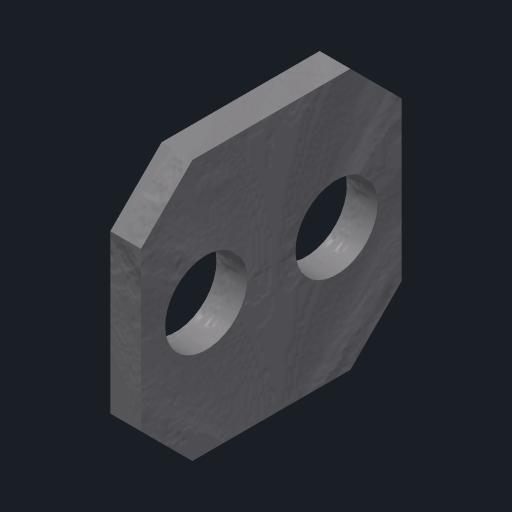
# Autodesk Inventor part: ACOPLE_TORNILLO_DOBLE
Saved by Autodesk Inventor 2024.3 (Build 283343000, 343)
## iProperties
Created: 2024-06-02
Part Number: ACOPLE_TORNILLO_DOBLE
Material: Steel, Mild, Welded
Document SubType Name: Modeling
Designer: Niler
Density: 7.85 g/cm^3
Appearance: Weld - Steel Mild
Author: Niler
Autodesk Inventor part; units mm, degrees
ref_plane "YZ Plane" through (0, 0, 0) normal (1, 0, 0) x (0, 1, 0)
ref_plane "XZ Plane" through (0, 0, 0) normal (0, 1, 0) x (-1, 0, 0)
ref_plane "XY Plane" through (0, 0, 0) normal (0, 0, 1) x (1, 0, 0)
sketch "Sketch1" plane through (0, 0, 0) normal (1, 0, 0) x (0, 1, 0)
  line L0 (-12.7, 12.7) -> (12.7, 12.7)
  line L1 (12.7, 12.7) -> (12.7, -12.7)
  line L2 (12.7, -12.7) -> (-12.7, -12.7)
  line L3 (-12.7, -12.7) -> (-12.7, 12.7)
  line L4 (-12.7, 12.7) -> (12.7, -12.7) construction
  line L5 (12.7, 12.7) -> (-12.7, -12.7) construction
  point P0 (0, 0)
  dimension "d0" = 25.4
  dimension "d1" = 25.4
  constraints: 12 end point, 2 midpoint, 2 parallel, 1 horizontal, 1 perpendicular
  measures "d0" distance of L1.end L2.end
  measures "d1" distance of L0.end L1.end
extrude "Extrusion1" add sketch "Sketch1" along normal blind 3
sketch "Sketch2" plane through (3, 0, 0) normal (1, 0, 0) x (0, 0, -1)
  line L0 (12.7, -12.7) -> (12.7, 12.7) projected
  line L1 (12.7, 12.7) -> (-12.7, 12.7) projected
  line L2 (-12.7, 12.7) -> (-12.7, -12.7) projected
  line L3 (-12.7, -12.7) -> (12.7, -12.7) projected
  line L4 (0, 12.7) -> (0, -12.7)
  circle A0 centre (-6.35, 0) radius 4
  line L5 (-11.85, 3.1754) -> (-6.35, 6.3509)
  line L6 (-6.35, 6.3509) -> (-0.85, 3.1754)
  line L7 (-0.85, 3.1754) -> (-0.85, -3.1754)
  line L8 (-0.85, -3.1754) -> (-6.35, -6.3509)
  line L9 (-6.35, -6.3509) -> (-11.85, -3.1754)
  line L10 (-11.85, -3.1754) -> (-11.85, 3.1754)
  circle A1 centre (6.35, 0) radius 4
  line L11 (11.85, 3.1754) -> (6.35, 6.3509)
  line L12 (6.35, 6.3509) -> (0.85, 3.1754)
  line L13 (0.85, 3.1754) -> (0.85, -3.1754)
  line L14 (0.85, -3.1754) -> (6.35, -6.3509)
  line L15 (6.35, -6.3509) -> (11.85, -3.1754)
  line L16 (11.85, -3.1754) -> (11.85, 3.1754)
  point P0 (0, 0)
  point P1 (0, 0)
  point P2 (-0.85, 0)
  point P3 (0.85, 0)
  dimension "d4" = 8
  dimension "d5" = 6.35
  dimension "d6" = 11
  constraints: 26 end point, 9 symmetric about line, 4 midpoint, 2 centre point, 2 coincident, 2 horizontal alignment, 14 other
  measures "d4" diameter of A0
  measures "d5" distance from line of L4 A0.centre
  measures "d6" distance between parallel lines of L7 L10
extrude "Extrusion2" cut sketch "Sketch2" against normal blind 3 contours A0 | A1
chamfer "Chamfer1" distance 5 angle 45 4 edges at (1.5, -12.7, -12.7) (1.5, -12.7, 12.7) (1.5, 12.7, 12.7) (1.5, 12.7, -12.7)
body "Solid1"
